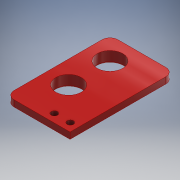
# Autodesk Inventor part: UltrasonicBase
Saved by Autodesk Inventor 2018.3 (Build 223284000, 284)
## iProperties
Created: 2020-03-24
Part Number: UltrasonicBase
Material: Generic
Document SubType Name: Modeling
Designer: Ivan
Density: 1 g/cm^3
Appearance: Default
Author: Ivan
Autodesk Inventor part; units mm, degrees
ref_plane "YZ Plane" through (0, 0, 0) normal (1, 0, 0) x (0, 1, 0)
ref_plane "XZ Plane" through (0, 0, 0) normal (0, 1, 0) x (-1, 0, 0)
ref_plane "XY Plane" through (0, 0, 0) normal (0, 0, 1) x (1, 0, 0)
sketch "Sketch1" plane through (0, 0, 0) normal (0, 0, 1) x (1, 0, 0)
  line L0 (0, 0) -> (-40, 0)
  line L1 (-40, 0) -> (-40, 65)
  line L2 (-40, 65) -> (0, 65)
  line L3 (0, 65) -> (0, 0)
  dimension "d0" = 40
  dimension "d1" = 65
  constraints: 8 end point, 2 parallel, 1 horizontal, 1 perpendicular
  measures "d0" distance between parallel lines of L3 L1
  measures "d1" distance between parallel lines of L0 L2
extrude "Extrusion1" add sketch "Sketch1" along normal blind 4
sketch "Sketch2" plane through (0, 0, 4) normal (0, 0, 1) x (1, 0, 0)
  circle A0 centre (-26, 51) radius 8
  circle A1 centre (-26, 25.117) radius 8
  line L0 (-40, 65) -> (-40, 0) projected
  line L1 (0, 65) -> (-40, 65) projected
  point P0 (0, 0)
  dimension "d4" = 16
  dimension "d5" = 16
  dimension "d6" = 14
  dimension "d7" = 14
  dimension "d8" = 25.883
  constraints: 2 centre point, 1 vertical alignment
  measures "d4" diameter of A0
  measures "d5" diameter of A1
  measures "d6" distance from line of L0 A0.centre
  measures "d7" distance from line of L1 A0.centre
  measures "d8" distance of A1.centre A0.centre
fillet "Fillet2" radius 5 2 edges at (-40, 65, 2) (0, 65, 2)
fillet "Fillet3" radius 5 1 edges at (-40, 0, 2)
sketch "Sketch4" plane through (0, 0, 4) normal (0, 0, 1) x (1, 0, 0)
  circle A0 centre (-5, 5.2) radius 2
  line L0 (0, 0) -> (0, 60) projected
  line L1 (-35, 0) -> (0, 0) projected
  circle A1 centre (-15, 5.2) radius 2
  dimension "d20" = 4
  dimension "d21" = 5
  dimension "d22" = 5.2
  dimension "d24" = 10
  dimension "d27" = 4
  constraints: 2 centre point, 1 horizontal alignment
  measures "d20" diameter of A0
  measures "d21" distance from line of L0 A0.centre
  measures "d22" distance from line of L1 A0.centre
  measures "d24" distance of A0.centre A1.centre
  measures "d27" diameter of A1
extrude "Extrusion5" cut sketch "Sketch4" against normal through all
sketch "Sketch6" plane through (0, 0, 0) normal (0, 0, -1) x (-1, 0, 0)
  circle A0 centre (26, 25.117) radius 8 projected
  circle A1 centre (26, 51) radius 8 projected
  circle A2 centre (26, 51) radius 11
  circle A3 centre (26, 25.117) radius 11
  point P0 (0, 0)
  dimension "d34" = 22
  dimension "d35" = 22
  constraints: 2 centre point, 2 coincident
  measures "d34" diameter of A2
  measures "d35" diameter of A3
extrude "Extrusion8" add sketch "Sketch6" along normal blind 3
fillet "Fillet4" radius 1 4 edges at (-15, 51, -3) (-18, 51, -3) (-15, 25.117, -3) (-18, 25.117, -3)
extrude "Extrusion9" cut sketch "Sketch2" against normal through all
equation "\"d5\" = d4"
equation "\"d27\" = d20"
body "Solid1"
